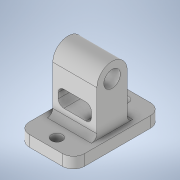
# Autodesk Inventor part: Peça2
Saved by Autodesk Inventor 2021 (Build 250183000, 183)
## iProperties
Created: 2022-02-01
Part Number: Peça2
Material: Genérico
Document SubType Name: Modeling
Designer: aluno
Density: 1 g/cm^3
Appearance: Padrão
Author: aluno
Autodesk Inventor part; units mm, degrees
ref_plane "YZ Plane" through (0, 0, 0) normal (1, 0, 0) x (0, 1, 0)
ref_plane "XZ Plane" through (0, 0, 0) normal (0, 1, 0) x (-1, 0, 0)
ref_plane "XY Plane" through (0, 0, 0) normal (0, 0, 1) x (1, 0, 0)
sketch "Esboço1" plane through (0, 0, 0) normal (0, 0, 1) x (1, 0, 0)
  line L0 (-80, -50) -> (80, -50)
  line L1 (80, -50) -> (80, 50)
  line L2 (80, 50) -> (-80, 50)
  line L3 (-80, 50) -> (-80, -50)
  line L4 (-80, -50) -> (80, 50) construction
  line L5 (80, -50) -> (-80, 50) construction
  point P0 (0, 0)
  dimension "d0" = 100
  dimension "d1" = 160
  constraints: 12 end point, 2 midpoint, 2 parallel, 1 horizontal, 1 perpendicular
  measures "d0" distance of L0.end L1.end
  measures "d1" distance of L0.start L0.end
extrude "Extrusão1" add sketch "Esboço1" along normal blind 20
sketch "Esboço2" plane through (0, 0, 20) normal (0, 0, 1) x (1, 0, 0)
  line L0 (-27.5, -40) -> (27.5, -40)
  line L1 (27.5, -40) -> (27.5, 40)
  line L2 (27.5, 40) -> (-27.5, 40)
  line L3 (-27.5, 40) -> (-27.5, -40)
  line L4 (-27.5, -40) -> (27.5, 40) construction
  line L5 (27.5, -40) -> (-27.5, 40) construction
  point P0 (0, 0)
  dimension "d4" = 55
  dimension "d5" = 80
  constraints: 12 end point, 2 midpoint, 2 parallel, 1 horizontal, 1 perpendicular
  measures "d4" distance of L2.end L1.end
  measures "d5" distance of L1.end L0.end
extrude "Extrusão2" add sketch "Esboço2" along normal blind 110
fillet "Arredondamento1" radius 27.5 2 edges at (-27.5, 0, 130) (27.5, 0, 130)
sketch "Esboço3" plane through (-27.5, -40, 20) normal (0, -1, 0) x (1, 0, 0)
  arc A0 (55, 82.5) -> (0, 82.5) centre (27.5, 82.5) ccw projected
  point P0 (27.5, -20)
  constraints: 1 coincident
hole "Furo1" at (0, -40, 102.5) direction (0, 1, 0) diameter 30 end through all
sketch "Esboço4" plane through (-27.5, -40, 20) normal (-1, 0, 0) x (0, 0, 1)
  line L0 (20, 70) -> (50, 70)
  line L1 (50, 70) -> (50, 10)
  line L2 (50, 10) -> (20, 10)
  line L3 (20, 10) -> (20, 70)
  line L4 (20, 70) -> (50, 10) construction
  line L5 (50, 70) -> (20, 10) construction
  line L6 (-20, -10) -> (-20, 90) projected
  line L7 (82.5, 80) -> (82.5, 0) projected
  point P0 (-20, 40)
  point P1 (35, 40)
  point P2 (35, 40)
  point P3 (82.5, 40)
  dimension "d18" = 60
  dimension "d19" = 55
  dimension "d20" = 30
  constraints: 12 end point, 4 midpoint, 2 parallel, 1 horizontal, 1 horizontal alignment, 1 perpendicular
  measures "d18" distance of L0.end L1.end
  measures "d19" distance from line of L6 point (35, 40)
  measures "d20" distance of L0.start L0.end
extrude "Extrusão3" cut sketch "Esboço4" against normal through all
sketch "Esboço5" plane through (0, 0, 20) normal (0, 0, 1) x (1, 0, 0)
  line L0 (-80, 50) -> (-80, -50) projected
  line L1 (-80, -50) -> (80, -50) projected
  line L2 (80, -50) -> (80, 50) projected
  point P0 (0, 0)
  point P1 (-60, 0)
  point P2 (60, 0)
  dimension "d23" = 20
  dimension "d24" = 50
  dimension "d25" = 20
  dimension "d26" = 50
  measures "d23" distance from line of L0 point (-60, 0)
  measures "d24" distance from line of L1 point (-60, 0)
  measures "d25" distance from line of L2 point (60, 0)
  measures "d26" distance from line of L1 point (60, 0)
hole "Furo2" at (-60, 0, 20) at (60, 0, 20) direction (0, 0, -1) diameter 20 end through all
fillet "Arredondamento2" radius 10 4 edges at (0, 30, 40) (0, -30, 70) (0, -30, 40) (0, 30, 70)
fillet "Arredondamento3" radius 10 2 edges at (-27.5, 0, 20) (27.5, 0, 20)
fillet "Arredondamento4" radius 20 4 edges at (80, -50, 10) (80, 50, 10) (-80, -50, 10) (-80, 50, 10)
equation "\"d8\" = 0.5 * d4"
equation "\"d24\" = 0.5 * d0"
equation "\"d26\" = 0.5 * d0"
